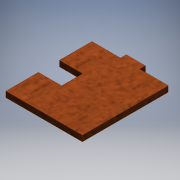
# Autodesk Inventor part: acople 3
Saved by Autodesk Inventor 2016 (Build 200138000, 138)
## iProperties
Created: 2016-08-02
Part Number: acople 3
Material: Madera (nogal)
Document SubType Name: Modeling
Designer: DanielFelipe
Density: 0.55 g/cm^3
Appearance: Nogal - Natural pulido
Mass: 2.79875 g
Surface Area: 39.934 cm^2
Volume: 5.08864 cm^3
Author: DanielFelipe
Autodesk Inventor part; units mm, degrees
ref_plane "YZ Plane" through (0, 0, 0) normal (1, 0, 0) x (0, 1, 0)
ref_plane "XZ Plane" through (0, 0, 0) normal (0, 1, 0) x (-1, 0, 0)
ref_plane "XY Plane" through (0, 0, 0) normal (0, 0, 1) x (1, 0, 0)
sketch "Boceto1" plane through (0, 0, 0) normal (0, 0, 1) x (1, 0, 0)
  line L0 (25, -3) -> (15, -3)
  line L1 (25, -3) -> (25, -6)
  line L2 (15, -6) -> (15, -3)
  line L3 (0, 0) -> (0, -3)
  line L4 (40, -6) -> (40, -3)
  line L5 (28.1623, -51) -> (8.1623, -51)
  line L6 (0, -6) -> (15, -6)
  line L7 (25, -6) -> (40, -6)
  line L8 (0, -6) -> (0, -51)
  line L9 (0, -51) -> (40, -51)
  line L10 (40, -51) -> (40, -6)
  line L11 (40, -6) -> (25, -6)
  line L12 (15, -6) -> (0, -6)
  point P0 (0, 0)
  constraints: 26 end point, 4 horizontal, 3 parallel, 2 perpendicular
extrude "Extrusión1" add sketch "Boceto1" along normal blind 3
sketch "Boceto2" plane through (0, 0, 3) normal (0, 0, 1) x (1, 0, 0)
  line L0 (25, -6) -> (25, -3) projected
  line L1 (25, -3) -> (15, -3) projected
  line L2 (15, -3) -> (15, -6) projected
  line L3 (15, -6) -> (0, -6) projected
  line L4 (0, -6) -> (0, -51) projected
  line L5 (0, -51) -> (40, -51) projected
  line L6 (40, -51) -> (40, -6) projected
  line L7 (40, -6) -> (25, -6) projected
  line L8 (40, -51) -> (40, -6)
  line L9 (0, -51) -> (40, -51)
  line L10 (0, -6) -> (0, -51)
  line L11 (15, -6) -> (0, -6)
  line L12 (15, -3) -> (15, -6)
  line L13 (40, -6) -> (25, -6)
  line L14 (25, -6) -> (25, -3)
  line L15 (25, -3) -> (15, -3)
  line L16 (9.8382, -32) -> (1.6623, -32)
  line L17 (9.8382, -31) -> (1.6623, -31)
  line L18 (1.1623, 19) -> (1.1623, 20)
  line L19 (10.1623, -31) -> (10.1623, -32)
  line L20 (9.8382, -30) -> (1.6623, -30)
  line L21 (9.8382, -29) -> (1.6623, -29)
  line L22 (1.1623, 21) -> (1.1623, 22)
  line L23 (10.1623, -29) -> (10.1623, -30)
  line L24 (9.8382, -25) -> (1.6623, -25)
  line L25 (1.1623, 25) -> (1.1623, 26)
  line L26 (9.8382, -26) -> (9.8382, -25)
  line L27 (0, -34) -> (12.1623, -34)
  line L28 (12.1623, -34) -> (12.1623, -23)
  line L29 (12.1623, -23) -> (0, -23)
  line L30 (0, -23) -> (0, -34)
  point P0 (0, 0)
  constraints: 46 end point, 3 vertical, 2 parallel, 1 horizontal, 1 perpendicular, 1 point on line, 6 other
extrude "Extrusión2" cut sketch "Boceto2" against normal blind 3 contours L4 L29 L28 L27
